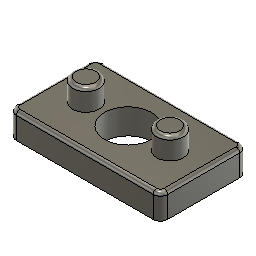
arri_to_smallhd (Autodesk Fusion 360 design; units mm, degrees)
Autodesk Fusion 360 part; units mm, degrees
sketch "Top" plane through (0, 0, 0) normal (0, 1, 0) x (1, 0, 0)
  line L0 (10.5, -6) -> (-10.5, -6)
  line L1 (-10.5, -6) -> (-10.5, 6)
  line L2 (-10.5, 6) -> (10.5, 6)
  line L3 (10.5, 6) -> (10.5, -6)
  line L4 (10.5, -6) -> (-10.5, 6) construction
  line L5 (-10.5, -6) -> (10.5, 6) construction
  line L6 (0, 0) -> (-10.5, 0) construction
  circle A0 centre (-7.5, 0) radius 1.6
  circle A1 centre (-5.842, 0) radius 1.8288
  line L7 (0, 0) -> (0, 6) construction
  circle A2 centre (7.5, 0) radius 1.6
  circle A3 centre (5.842, 0) radius 1.8288
  circle A4 centre (0, 0) radius 3.25
  dimension "d1" = 21
  dimension "d2" = 12
  dimension "d3" = 3.2
  dimension "d4" = 7.5
  dimension "d5" = 3.6576
  dimension "d6" = 5.842
  dimension "d14" = 6.5
  constraint horizontal L0
  constraint perpendicular L0 L1
  constraint parallel L0 L2
  constraint parallel L1 L3
  constraint coincident L4 L6.start
  constraint coincident L5 L6.start
  constraint coincident L6.start L7.start
  constraint midpoint L1 L6.end
  constraint coincident L6 A0.centre
  constraint coincident L6 A1.centre
  constraint midpoint L2 L7.end
  constraint symmetric A0 L7 A2
  constraint symmetric A1 L7 A3
  measures "d1" distance of L1.end L2.end
  measures "d2" distance of L0.end L1.end
  measures "d3" diameter of A0
  measures "d4" distance of L6.start A0.centre
  measures "d5" diameter of A1
  measures "d6" distance of L6.start A1.centre
  measures "d14" diameter of A4
extrude "Extrude1" add sketch "Top" along normal blind 3.5 contours L0 L1 L2 L3 | A0 A1 | A0 A1 | A0 A1 | A2 A3 | A2 A3 | A2 A3
extrude "Extrude2" add sketch "Top" along normal blind 3 from surface at 3.5 contours A0 A1 | A0 A1 | A2 A3 | A2 A3 picked at (-7.0773, 0) picked at (-4.6486, 0.0888) picked at (7.0808, -0.1615) picked at (4.6486, 0.0888)
extrude "Extrude3" cut sketch "Top" along normal blind 3 contours A0 A1 | A0 A1 | A2 A3 | A2 A3 picked at (-7.0773, 0) picked at (-8.1426, -0.0385) picked at (8.1364, -0.1564) picked at (7.0808, -0.1615)
fillet "Fillet1" radius 0.5 4 edges at (-10.5, 3.5, 0) (0, 3.5, -6) (10.5, 3.5, 0) (0, 3.5, 6)
fillet "Fillet2" radius 1 8 edges at (-10.5, 1.5, 6) (-10.3536, 3.3536, 5.8536) (10.5, 1.5, 6) (10.3536, 3.3536, 5.8536) (10.5, 1.5, -6) (10.3536, 3.3536, -5.8536) (-10.5, 1.5, -6) (-10.3536, 3.3536, -5.8536)
fillet "Fillet3" radius 0.5 2 edges at (-7.547, 6.5, 0.6613) (4.137, 6.5, 0.6613)
fillet "Fillet4" radius 0.5 2 edges at (-8.9917, 0, 0.5786) (6.0083, 0, 0.5786)
equation "d4 = ( 15 / 2 ) * 1 mm"
named bodies: "ARRI-to-SmallHD adapter"
